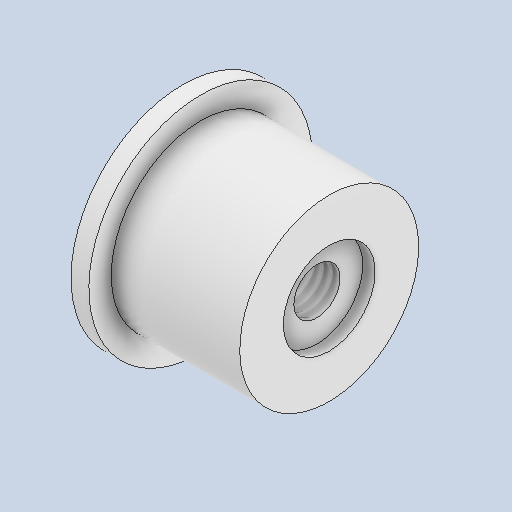
# Autodesk Inventor part: SpringCompensation_Innside_SupportPart
Saved by Autodesk Inventor 2024 (Build 280153000, 153)
## iProperties
Created: 2022-10-13
Part Number: SpringCompensation_Innside_SupportPart
Material: PBT-Kunststoff
Document SubType Name: Modeling
Designer: alexw
Density: 1.31 g/cm^3
Appearance: Glatt - Weiß
Mass: 3.40038 g
Surface Area: 14.6424 cm^2
Volume: 2.59571 cm^3
Author: alexw
Autodesk Inventor part; units mm, degrees
ref_plane "YZ Plane" through (0, 0, 0) normal (1, 0, 0) x (0, 1, 0)
ref_plane "XZ Plane" through (0, 0, 0) normal (0, 1, 0) x (-1, 0, 0)
ref_plane "XY Plane" through (0, 0, 0) normal (0, 0, 1) x (1, 0, 0)
sketch "Skizze1" plane through (0, 0, 0) normal (0, 0, 1) x (1, 0, 0)
  line L0 (0, 0) -> (0, 10)
  line L1 (0, 10) -> (1.6, 10)
  line L2 (1.6, 10) -> (1.6, 8)
  line L3 (1.6, 8) -> (13.1, 8)
  line L4 (13.1, 8) -> (13.1, 4)
  line L5 (0, 0) -> (12, 0)
  line L6 (13.1, 4) -> (12, 4)
  line L7 (12, 4) -> (12, 0)
  dimension "d0" = 16
  dimension "d1" = 20
  dimension "d2" = 11.5
  dimension "d3" = 1.6
  dimension "d12" = 8
  dimension "d13" = 10.4
  constraints: 16 end point, 5 perpendicular, 2 horizontal, 1 vertical
  measures "d0" diameter of L3 L5
  measures "d1" diameter of L1 L5
  measures "d2" distance between parallel lines of L4 L2
  measures "d3" distance between parallel lines of L0 L2
  measures "d12" diameter of L6 L5
  measures "d13" distance between parallel lines of L2 L7
revolve "Umdrehung1" add sketch "Skizze1" angle 360 about axis through (0, 0, 0) along (1, 0, 0)
sketch "Skizze2" plane through (0, 0, 0) normal (-1, 0, 0) x (0, 0, 1)
  point P0 (0, 0)
  point P1 (0, 0)
  constraints: 1 coincident
hole "Bohrung1" at (0, 0, 0) direction (1, 0, 0) diameter 4.134 depth 14.2 tip angle 118 thread size "M5x0.8" class "6H" standard "ISO Metric profile"
feature "Verdickung1" [suppressed]
thicken "Verdickung2" operation add thickness 0.1 both sides no extend neighbours yes toward (0, 0.9870503, -0.1604113) faces at (12.7333, 3.9482, -0.6416)
